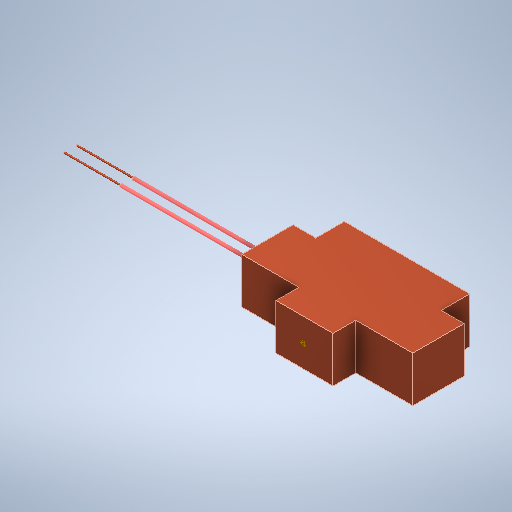
# Autodesk Inventor part: AlN_thermal_contact
Saved by Autodesk Inventor 2025 (Build 290162000, 162)
## iProperties
Created: 2024-04-25
Part Number: AlN_thermal_contact
Material: Copper
Document SubType Name: Modeling
Designer: warke
Density: 8.94 g/cm^3
Appearance: Copper - Satin
Mass: 1.2696 g
Surface Area: 4.90867 cm^2
Volume: 0.399246 cm^3
Author: warke
Autodesk Inventor part; units mm, degrees
ref_plane "YZ Plane" through (0, 0, 0) normal (1, 0, 0) x (0, 1, 0)
ref_plane "XZ Plane" through (0, 0, 0) normal (0, 1, 0) x (-1, 0, 0)
ref_plane "XY Plane" through (0, 0, 0) normal (0, 0, 1) x (1, 0, 0)
sketch "Sketch1" plane through (0, 0, 0) normal (0, 1, 0) x (-1, 0, 0)
  line L0 (-7.5, 15) -> (7.5, 15)
  line L1 (7.5, 15) -> (7.5, -15)
  line L2 (7.5, -15) -> (-7.5, -15)
  line L3 (-7.5, -15) -> (-7.5, 15)
  line L4 (-7.5, 15) -> (7.5, -15) construction
  line L5 (7.5, 15) -> (-7.5, -15) construction
  point P0 (0, 0)
  dimension "d0" = 15
  dimension "d1" = 30
  constraints: 12 end point, 2 midpoint, 2 parallel, 1 horizontal, 1 perpendicular
  measures "d0" distance of L1.end L2.end
  measures "d1" distance of L0.end L1.end
extrude "Extrusion1" add sketch "Sketch1" along normal blind 4
chamfer "Chamfer1" distance 2.5 distance2 1 1 edges at (7.5, 2, -15) measured on face at (7.5, 1.3333, 5)
chamfer "Chamfer2" distance 1 distance2 2.5 1 edges at (-7.5, 2, -15) measured on face at (1.8333, 2.6667, -15)
sketch "Sketch3" plane through (0, 0, 0) normal (0, -1, 0) x (1, 0, 0)
  line L0 (0, 0) -> (4, 0)
  line L1 (0, 0) -> (-4, 0)
  dimension "d14" = 4
  dimension "d15" = 4
  constraints: 4 end point, 2 coincident, 2 horizontal
  measures "d14" distance of L0.start L0.end
  measures "d15" distance of L0.start L1.end
hole "Hole1" at (4, 0, 0) at (-4, 0, 0) direction (0, 1, 0) diameter 2.1565 end through all thread size "4-40 UNC" class "2B" standard "ANSI Unified Screw Threads"
sketch "Sketch4" plane through (0, 0, 0) normal (0, -1, 0) x (1, 0, 0)
  line L0 (7.5, 15) -> (7.5, -12.5) projected
  line L1 (7.5, -12.5) -> (7.5, -7.5)
  line L2 (7.5, -7.5) -> (2.5, -7.5)
  line L3 (2.5, -7.5) -> (2.5, -5.5)
  line L4 (2.5, -5.5) -> (-2.5, -5.5)
  line L5 (-2.5, -5.5) -> (-2.5, -7.5)
  line L6 (-2.5, -7.5) -> (-7.5679, -7.5)
  line L7 (-7.5679, -7.5) -> (-7.5679, -12.5)
  line L8 (6.5, -15) -> (-6.5, -15) projected
  line L9 (-7.5679, -12.5) -> (-6.5, -15)
  line L10 (7.5, -12.5) -> (6.5, -15) projected
  line L11 (-6.5, -15) -> (6.5, -15)
  line L12 (6.5, -15) -> (7.5, -12.5)
  point P0 (0, 0)
  dimension "d23" = 5
  dimension "d24" = 5
  dimension "d25" = 2
  dimension "d26" = 5
  constraints: 20 end point, 5 perpendicular, 3 point on line, 1 collinear, 1 parallel
  measures "d23" distance of L0.end L1.end
  measures "d24" distance of L1.end L2.end
  measures "d25" distance of L2.end L3.end
  measures "d26" distance of L3.end L4.end
split body "Split1" sketch "Sketch4" result one side removed curves L2 L3 L4 L5 L6 L7 L9 L11 L12 L1 removed pieces at (1.1663, 0.5, 10.3182)
sketch "Sketch5" plane through (-7.5, 0, -12.5) normal (-1, 0, 0) x (0, 0, 1)
  line L0 (0, 0) -> (0, 4) projected
  line L1 (-2.5, 4) -> (-2.5, 0) projected
  line L2 (0, 0) -> (-2.5, 0)
  line L3 (-2.5, 0) -> (-2.5, 4)
  line L4 (-2.5, 4) -> (0, 4)
  line L5 (0, 4) -> (0, 0)
  point P0 (12.5, 0)
  constraints: 8 end point, 2 parallel, 1 horizontal, 1 perpendicular
extrude "Extrusion3" cut sketch "Sketch5" against normal blind 2
sketch "Sketch6" plane through (7.5, 0, -12.5) normal (1, 0, 0) x (0, 0, -1)
  line L0 (0, 4) -> (0, 0) projected
  line L1 (2.5, 0) -> (2.5, 4) projected
  line L2 (0, 4) -> (2.5, 4)
  line L3 (2.5, 4) -> (2.5, 0)
  line L4 (2.5, 0) -> (0, 0)
  line L5 (0, 0) -> (0, 4)
  point P0 (-12.5, 0)
  constraints: 8 end point, 2 parallel, 1 horizontal, 1 perpendicular
extrude "Extrusion4" cut sketch "Sketch6" against normal blind 2
hole "Hole2" at (-7.5, 2, -10) direction (1, 0, 0) diameter 2.5 depth 7.5
sketch "Sketch7" plane through (-7.5, 0, -12.5) normal (0, 0, -1) x (-1, 0, 0)
  line L0 (0, 0) -> (0, 4) projected
  line L1 (-2, 4) -> (0, 4) projected
  line L2 (-2, 4) -> (-2, 0) projected
  line L3 (0, 0) -> (-2, 0) projected
  point P0 (-7.5, 0)
extrude "Extrusion5" cut sketch "Sketch7" against normal blind 0.5
sketch "Sketch8" plane through (7.5, 0, -12.5) normal (0, 0, -1) x (-1, 0, 0)
  line L0 (2, 0) -> (0, 0) projected
  line L1 (0, 4) -> (0, 0) projected
  line L2 (2, 0) -> (0, 0) projected
  line L3 (2, 0) -> (2, 4) projected
  line L4 (0, 4) -> (2, 4) projected
  point P0 (7.5, 0)
extrude "Extrusion6" cut sketch "Sketch8" against normal blind 0.5
sketch "Sketch9" plane through (-5.5, 0, -12.5) normal (-1, 0, 0) x (0, 0, 1)
  line L0 (-2.5, 0) -> (-2.5, 4) projected
  line L1 (-2.5, 2) -> (-1.013, 2)
  point P0 (12.5, 0)
  dimension "d44" = 1.487
  constraints: 2 end point, 1 horizontal, 1 midpoint
  measures "d44" distance of L1.start L1.end
hole "Hole3" [suppressed]
sketch "Sketch10" plane through (5.5, 0, -12.5) normal (1, 0, 0) x (0, 0, -1)
  circle A0 centre (1.013, 2) radius 0.5953 projected
  point P0 (-12.5, 0)
  constraints: 1 coincident
hole "Hole4" [suppressed]
sketch "Sketch11" plane through (-5.5, 0, -15) normal (0, 0, -1) x (-1, 0, 0)
  line L0 (-11, 4) -> (-11, 0) projected
  line L1 (-11, 0) -> (0, 0) projected
  line L2 (-11, 4) -> (0, 4)
  line L3 (0, 4) -> (0, 0)
  line L4 (0, 0) -> (-11, 0)
  line L5 (-11, 0) -> (-11, 4)
  point P0 (-5.5, 0)
  constraints: 8 end point, 2 parallel, 1 horizontal, 1 perpendicular
extrude "Extrusion7" cut sketch "Sketch11" against normal blind 0.5
sketch "Sketch12" plane through (0, 2, -10) normal (-1, 0, 0) x (0, 0, 1)
  circle A0 centre (-0.55, 0) radius 0.15
  circle A1 centre (0.55, 0) radius 0.15
  point P0 (10, -2)
  dimension "d63" = 0.3
  dimension "d64" = 0.3
  constraints: 2 centre point, 2 coincident
  measures "d63" diameter of A0
  measures "d64" diameter of A1
extrude "Extrusion8" add sketch "Sketch12" along normal blind 25
sketch "Sketch13" plane through (-25, 2, -10.55) normal (-1, 0, 0) x (0, 0, 1)
  circle A0 centre (0, 0) radius 0.15 projected
  circle A1 centre (0, 0) radius 0.075
  circle A2 centre (1.1, 0) radius 0.15 projected
  circle A3 centre (1.1, 0) radius 0.075
  circle A4 centre (0, 0) radius 0.15 projected
  circle A5 centre (1.1, 0) radius 0.15 projected
  point P0 (10.55, -2)
  dimension "d67" = 0.15
  dimension "d68" = 0.15
  constraints: 2 centre point, 2 coincident
  measures "d67" diameter of A1
  measures "d68" diameter of A3
extrude "Extrusion9" cut sketch "Sketch13" against normal blind 5
body "Solid1"
